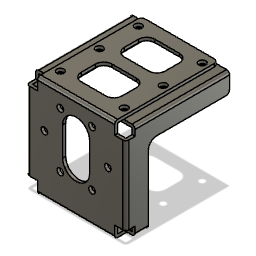
move_base_motor_holder (Autodesk Fusion 360 design; units mm, degrees)
Autodesk Fusion 360 part; units mm, degrees
sketch "スケッチ10" plane through (0, 0, 0) normal (0, 0, 1) x (1, 0, 0)
  line L0 (-18.8, 0) -> (18.8, 0)
  line L1 (18.8, 0) -> (18.8, -4.5)
  line L2 (18.8, -4.5) -> (22.8, -4.5)
  line L3 (22.8, -4.5) -> (22.8, -42.5)
  line L4 (22.8, -42.5) -> (18.8, -42.5)
  line L5 (18.8, -42.5) -> (18.8, -47)
  line L6 (18.8, -47) -> (-18.8, -47)
  line L7 (-18.8, -47) -> (-18.8, -42.5)
  line L8 (-18.8, -42.5) -> (-22.8, -42.5)
  line L9 (-22.8, -42.5) -> (-22.8, -4.5)
  line L10 (-22.8, -4.5) -> (-18.8, -4.5)
  line L11 (-18.8, -4.5) -> (-18.8, 0)
  dimension "d76" = 37.6
  dimension "d77" = 4.5
  dimension "d78" = 38
  dimension "d79" = 4.5
  dimension "d80" = 4
  dimension "d81" = 4
  constraint horizontal L0
  constraint perpendicular L0 L1
  constraint perpendicular L1 L2
  constraint perpendicular L2 L3
  constraint perpendicular L1 L4
  constraint perpendicular L2 L5
  constraint perpendicular L5 L6
  constraint perpendicular L6 L7
  constraint perpendicular L7 L8
  constraint perpendicular L8 L9
  constraint perpendicular L9 L10
  constraint perpendicular L8 L11
  constraint coincident L0.start L11.end
  constraint midpoint origin L0
  constraint collinear L1 L5
  constraint collinear L7 L11
  constraint collinear L2 L10
  constraint collinear L4 L8
  measures "d76" distance of L0.start L0.end
  measures "d77" distance of L0.end L1.end
  measures "d78" distance of L2.end L3.end
  measures "d79" distance of L4.end L5.end
  measures "d80" distance of L1.end L2.end
  measures "d81" distance of L9.end L10.end
extrude "押し出し8" add sketch "スケッチ10" along normal blind 1.5
sketch "スケッチ11" plane through (0, 0, 0) normal (0, 1, 0) x (-1, 0, 0)
  line L0 (-18.8, 0) -> (18.8, 0)
  line L1 (18.8, 0) -> (18.8, 1.5)
  line L2 (18.8, 1.5) -> (-18.8, 1.5)
  line L3 (-18.8, 1.5) -> (-18.8, 0)
  line L4 (18.8, 1.5) -> (-18.8, 1.5)
  line L5 (-18.8, 1.5) -> (-18.8, -49.2)
  line L6 (-18.8, -49.2) -> (18.8, -49.2)
  line L7 (18.8, -49.2) -> (18.8, 1.5)
  line L8 (-10, -7) -> (10, -7)
  line L9 (10, -7) -> (10, -22)
  line L10 (10, -22) -> (-10, -22)
  line L11 (-10, -22) -> (-10, -7)
  line L12 (-10, -28) -> (10, -28)
  line L13 (10, -28) -> (10, -43)
  line L14 (10, -43) -> (-10, -43)
  line L15 (-10, -43) -> (-10, -28)
  point P0 (0, -7)
  dimension "d84" = 50.7
  dimension "d172" = 7
  dimension "d173" = 15
  dimension "d174" = 6
  dimension "d175" = 15
  dimension "d176" = 20
  constraint horizontal L4
  constraint vertical L5
  constraint horizontal L6
  constraint vertical L7
  constraint coincident L1.end L2.start
  constraint coincident L2.end L3.start
  constraint horizontal L8
  constraint vertical L9
  constraint horizontal L10
  constraint vertical L11
  constraint horizontal L12
  constraint vertical L13
  constraint horizontal L14
  constraint vertical L15
  constraint midpoint L8 P0
  constraint collinear L11 L15
  constraint collinear L9 L13
  constraint vertical origin P0
  measures "d84" distance of L2.end L5.end
  measures "d172" distance of origin L8
  measures "d173" distance of L8.end L9.end
  measures "d174" distance of L10 L12
  measures "d175" distance of L12.end L13.end
  measures "d176" distance of L13.end L14.end
extrude "押し出し9" add sketch "スケッチ11" along normal blind 1.5
sketch "スケッチ17" plane through (0, 1.5, 0) normal (0, 1, 0) x (-1, 0, 0)
  line L0 (18.8, -49.2) -> (18.8, 1.5)
  line L1 (18.8, 1.5) -> (-18.8, 1.5)
  line L2 (-18.8, 1.5) -> (-18.8, -49.2)
  line L3 (-18.8, -49.2) -> (18.8, -49.2)
  line L4 (15.6, -6.4) -> (-15.6, -6.4)
  line L5 (-15.6, -6.4) -> (-15.6, -44.5)
  line L6 (-15.6, -44.5) -> (15.6, -44.5)
  line L7 (15.6, -44.5) -> (15.6, -6.4)
  line L8 (15.6, -25.45) -> (-15.6, -25.45)
  line L9 (10, -22) -> (-10, -22)
  line L10 (-10, -22) -> (-10, -7)
  line L11 (-10, -7) -> (10, -7)
  line L12 (10, -7) -> (10, -22)
  line L13 (10, -43) -> (-10, -43)
  line L14 (-10, -43) -> (-10, -28)
  line L15 (-10, -28) -> (10, -28)
  line L16 (10, -28) -> (10, -43)
  point P0 (0, -6.4)
  dimension "d112" = 7.9
  dimension "d113" = 31.2
  dimension "d114" = 19.05
  dimension "d115" = 19.05
  constraint horizontal L4
  constraint vertical L5
  constraint horizontal L6
  constraint vertical L7
  constraint midpoint L4 P0
  constraint vertical origin P0
  constraint coincident L7 L8.start
  constraint coincident L5 L8.end
  constraint perpendicular L5 L8
  measures "d112" distance of L1 L4
  measures "d113" distance of L4.start L4.end
  measures "d114" distance of L4 L8
  measures "d115" distance of L6 L8
hole "穴5" at (-15.6, 1.5, -44.5) at (15.6, 1.5, -44.5) at (15.6, 1.5, -25.45) at (-15.6, 1.5, -25.45) at (-15.6, 1.5, -6.4) at (15.6, 1.5, -6.4) direction (0, -1, 0) diameter 3.5 end through all
sketch "スケッチ12" plane through (0, -47, 0) normal (0, -1, 0) x (1, 0, 0)
  line L0 (-18.8, 0) -> (18.8, 0)
  line L1 (18.8, 0) -> (18.8, 1.5)
  line L2 (18.8, 1.5) -> (-18.8, 1.5)
  line L3 (-18.8, 1.5) -> (-18.8, 0)
  line L4 (18.8, 1.5) -> (-18.8, 1.5)
  line L5 (-18.8, 1.5) -> (-18.8, -9.5)
  line L6 (-18.8, -9.5) -> (18.8, -9.5)
  line L7 (18.8, -9.5) -> (18.8, 1.5)
  dimension "d87" = 11
  constraint horizontal L4
  constraint vertical L5
  constraint horizontal L6
  constraint vertical L7
  constraint coincident L1.end L2.start
  constraint coincident L2.end L3.start
  measures "d87" distance of L4 L6
extrude "押し出し10" add sketch "スケッチ12" along normal blind 1.5
sketch "スケッチ18" plane through (0, -48.5, 0) normal (0, -1, 0) x (1, 0, 0)
  line L0 (18.8, -9.5) -> (18.8, 1.5)
  line L1 (18.8, 1.5) -> (-18.8, 1.5)
  line L2 (-18.8, 1.5) -> (-18.8, -9.5)
  line L3 (-18.8, -9.5) -> (18.8, -9.5)
  line L4 (15.6, -6.4) -> (-15.6, -6.4)
  point P0 (0, -6.4)
  dimension "d119" = 7.9
  dimension "d120" = 31.2
  constraint horizontal L4
  constraint midpoint L4 P0
  constraint vertical origin P0
  measures "d119" distance of L1 L4
  measures "d120" distance of L4.start L4.end
hole "穴6" at (15.6, -48.5, -6.4) at (-15.6, -48.5, -6.4) direction (0, 1, 0) diameter 3.5 depth 1.5 tip angle 118
sketch "スケッチ13" plane through (22.8, 0, 0) normal (1, 0, 0) x (0, 0, -1)
  line L0 (0, -42.5) -> (0, -4.5)
  line L1 (0, -4.5) -> (-1.5, -4.5)
  line L2 (-1.5, -4.5) -> (-1.5, -42.5)
  line L3 (-1.5, -42.5) -> (0, -42.5)
  line L4 (-1.5, -4.5) -> (3, -4.5)
  line L5 (3, -4.5) -> (3, -1.55)
  line L6 (3, -1.55) -> (49.2, -1.55)
  line L7 (9.5, -45.45) -> (3, -45.45)
  line L8 (3, -45.45) -> (3, -42.5)
  line L9 (3, -42.5) -> (-1.5, -42.5)
  line L10 (-1.5, -42.5) -> (-1.5, -4.5)
  line L11 (49.2, -1.55) -> (49.2, -9.5)
  line L12 (49.2, -9.5) -> (9.5, -9.5)
  line L13 (9.5, -9.5) -> (9.5, -45.45)
  dimension "d90" = 4.5
  dimension "d92" = 2.95
  dimension "d93" = 2.95
  dimension "d109" = 46.2
  dimension "d110" = 7.95
  dimension "d111" = 6.5
  constraint coincident L1.end L2.start
  constraint perpendicular L0 L4
  constraint perpendicular L4 L5
  constraint perpendicular L0 L6
  constraint perpendicular L7 L8
  constraint coincident L2.end L3.start
  constraint collinear L5 L8
  constraint perpendicular L6 L11
  constraint perpendicular L11 L12
  constraint perpendicular L12 L13
  constraint coincident L7.start L13.end
  measures "d90" distance of L1.end L4.end
  measures "d92" distance of L4.end L5.end
  measures "d93" distance of L7 L9
  measures "d109" distance of L5.end L6.end
  measures "d110" distance of L6.end L11.end
  measures "d111" distance of L7.start L7.end
extrude "押し出し11" add sketch "スケッチ13" along normal blind 1.5
sketch "スケッチ20" plane through (-22.8, 0, 0) normal (-1, 0, 0) x (0, 0, 1)
  line L0 (0, -4.5) -> (0, -42.5)
  line L1 (0, -42.5) -> (1.5, -42.5)
  line L2 (1.5, -42.5) -> (1.5, -4.5)
  line L3 (1.5, -4.5) -> (0, -4.5)
  line L4 (1.5, -4.5) -> (-3, -4.5)
  line L5 (-3, -4.5) -> (-3, -1.55)
  line L6 (-3, -1.55) -> (-49.2, -1.55)
  line L7 (-49.2, -1.55) -> (-49.2, -9.5)
  line L8 (-49.2, -9.5) -> (-9.5, -9.5)
  line L9 (-9.5, -9.5) -> (-9.5, -45.45)
  line L10 (-9.5, -45.45) -> (-3, -45.45)
  line L11 (-3, -45.45) -> (-3, -42.5)
  line L12 (-3, -42.5) -> (1.5, -42.5)
  line L13 (1.5, -42.5) -> (1.5, -4.5)
  point P0 (-3, -4.5)
  point P1 (-3, -1.55)
  point P2 (-49.2, -1.55)
  point P3 (-49.2, -9.5)
  point P4 (-9.5, -9.5)
  point P5 (-9.5, -45.45)
  point P6 (-3, -42.5)
  constraint coincident L2.end L3.start
  constraint perpendicular L0 L4
  constraint perpendicular L4 L5
  constraint perpendicular L5 L6
  constraint perpendicular L6 L7
  constraint perpendicular L5 L8
  constraint perpendicular L8 L9
  constraint perpendicular L9 L10
  constraint perpendicular L10 L11
  constraint coincident L1.end L2.start
  constraint coincident P0 L4.end
  constraint coincident L6 P1
  constraint coincident P2 L6.end
  constraint coincident P3 L7.end
  constraint coincident L9 P4
  constraint coincident P5 L9.end
  constraint coincident P6 L11.end
extrude "押し出し14" add sketch "スケッチ20" along normal blind 1.5
sketch "スケッチ14" plane through (0, -1.55, 0) normal (0, 1, 0) x (-1, 0, 0)
  line L0 (-22.8, -49.2) -> (-22.8, -3)
  line L1 (-22.8, -3) -> (-24.3, -3)
  line L2 (-24.3, -3) -> (-24.3, -49.2)
  line L3 (-24.3, -3) -> (-11.3, -3)
  line L4 (-11.3, -3) -> (-11.3, -49.2)
  line L5 (-11.3, -49.2) -> (-24.3, -49.2)
  line L6 (-24.3, -49.2) -> (-24.3, -3)
  line L7 (-24.3, -49.2) -> (-22.8, -49.2)
  dimension "d96" = 13
  constraint horizontal L3
  constraint vertical L4
  constraint horizontal L5
  constraint vertical L6
  constraint coincident L1.end L2.start
  constraint coincident L2.end L5.end
  measures "d96" distance of L4.end L2.end
extrude "押し出し12" add sketch "スケッチ14" along normal blind 1.5
sketch "スケッチ19" plane through (0, -0.05, 0) normal (0, 1, 0) x (-1, 0, 0)
  line L0 (-11.3, -49.2) -> (-11.3, -3)
  line L1 (-11.3, -3) -> (-24.3, -3)
  line L2 (-24.3, -3) -> (-24.3, -49.2)
  line L3 (-24.3, -49.2) -> (-11.3, -49.2)
  line L4 (-15.6, -6.4) -> (-15.6, -44.5)
  line L5 (18.8, 1.5) -> (-18.8, 1.5)
  point P0 (-15.6, -25.45)
  dimension "d124" = 15.6
  dimension "d125" = 7.9
  dimension "d126" = 38.1
  constraint parallel L0 L4
  constraint midpoint L4 P0
  measures "d124" distance of origin L4
  measures "d125" distance of L4.start L5
  measures "d126" distance of L4.start L4.end
hole "穴7" at (15.6, -0.05, -44.5) at (15.6, -0.05, -25.45) at (15.6, -0.05, -6.4) direction (0, -1, 0) diameter 3 depth 1.5 tip angle 118
sketch "スケッチ15" plane through (0, -45.45, 0) normal (0, -1, 0) x (1, 0, 0)
  line L0 (22.8, -3) -> (22.8, -9.5)
  line L1 (24.3, -9.5) -> (24.3, -3)
  line L2 (24.3, -3) -> (22.8, -3)
  line L3 (24.3, -3) -> (11.3, -3)
  line L4 (11.3, -3) -> (11.3, -9.5)
  line L5 (11.3, -9.5) -> (24.3, -9.5)
  line L6 (24.3, -9.5) -> (24.3, -3)
  line L7 (22.8, -9.5) -> (24.3, -9.5)
  line L8 (18.8, 1.5) -> (-18.8, 1.5)
  point P0 (15.6, -6.4)
  dimension "d99" = 13
  dimension "d134" = 7.9
  dimension "d135" = 15.6
  constraint horizontal L3
  constraint vertical L4
  constraint horizontal L5
  constraint vertical L6
  constraint coincident L1.end L2.start
  constraint coincident L1.start L5.end
  measures "d99" distance of L4 L6
  measures "d134" distance of P0 L8
  measures "d135" horizontal distance of origin P0
extrude "押し出し13" add sketch "スケッチ15" along normal blind 1.5
hole "穴8" at (15.6, -45.45, -6.4) direction (0, -1, 0) diameter 3 end through all
sketch "スケッチ21" plane through (0, -1.55, 0) normal (0, 1, 0) x (-1, 0, 0)
  line L0 (22.8, -3) -> (22.8, -49.2)
  line L1 (22.8, -49.2) -> (24.3, -49.2)
  line L2 (24.3, -49.2) -> (24.3, -3)
  line L3 (24.3, -3) -> (22.8, -3)
  line L4 (24.3, -3) -> (11.3, -3)
  line L5 (11.3, -3) -> (11.3, -49.2)
  line L6 (11.3, -49.2) -> (24.3, -49.2)
  line L7 (24.3, -49.2) -> (24.3, -3)
  line L8 (15.6, -6.4) -> (15.6, -44.5)
  line L9 (18.8, 1.5) -> (-18.8, 1.5)
  point P0 (15.6, -25.45)
  dimension "d139" = 13
  dimension "d140" = 7.9
  dimension "d141" = 15.6
  dimension "d142" = 38.1
  constraint horizontal L4
  constraint vertical L5
  constraint horizontal L6
  constraint vertical L7
  constraint coincident L2.end L3.start
  constraint coincident L1.end L2.start
  constraint vertical L8
  constraint midpoint L8 P0
  measures "d139" distance of L5 L7
  measures "d140" distance of L8.start L9
  measures "d141" horizontal distance of origin L8.start
  measures "d142" distance of L8.start L8.end
extrude "押し出し15" add sketch "スケッチ21" along normal blind 1.5
hole "穴9" at (-15.6, -1.55, -44.5) at (-15.6, -1.55, -25.45) at (-15.6, -1.55, -6.4) direction (0, 1, 0) diameter 3 end through all
sketch "スケッチ22" plane through (0, -45.45, 0) normal (0, -1, 0) x (1, 0, 0)
  line L0 (-22.8, -9.5) -> (-22.8, -3)
  line L1 (-22.8, -3) -> (-24.3, -3)
  line L2 (-24.3, -3) -> (-24.3, -9.5)
  line L3 (-24.3, -9.5) -> (-22.8, -9.5)
  line L4 (-24.3, -3) -> (-11.3, -3)
  line L5 (-11.3, -3) -> (-11.3, -9.5)
  line L6 (-11.3, -9.5) -> (-24.3, -9.5)
  line L7 (-24.3, -9.5) -> (-24.3, -3)
  line L8 (18.8, 1.5) -> (-18.8, 1.5)
  point P0 (-15.6, -6.4)
  dimension "d148" = 13
  dimension "d149" = 7.9
  dimension "d150" = 15.6
  constraint horizontal L4
  constraint vertical L5
  constraint horizontal L6
  constraint vertical L7
  constraint coincident L1.end L2.start
  constraint coincident L2.end L3.start
  measures "d148" distance of L5 L7
  measures "d149" distance of P0 L8
  measures "d150" horizontal distance of origin P0
extrude "押し出し16" add sketch "スケッチ22" along normal blind 1.5
hole "穴10" at (-15.6, -45.45, -6.4) direction (0, -1, 0) diameter 3 end through all
thread "ねじ1" "ISO Metric profile 3.0 M3x0.5 6H" major diameter 3.086 minor diameter 2.529 pitch 0.5 angle 60 resizes the face on face at (15.7494, -1.05, -4.9075) on face at (16.9348, -1.05, -45.1843) on face at (-14.2327, -1.05, -43.8831) on face at (15.7494, -1.05, -23.9575) on face at (-15.4506, -0.55, -7.8925) on face at (-15.5252, -1.05, -26.9481) on face at (15.7494, -46.45, -4.9075) on face at (-15.4506, -46.45, -4.9075)
fillet "フィレット3" radius 1.5 8 edges at (0, 1.5, 1.5) (-24.3, -0.05, -26.1) (24.3, -0.05, -26.1) (24.3, -23.5, 1.5) (-24.3, -23.5, 1.5) (0, -48.5, 1.5) (-24.3, -46.95, -6.25) (24.3, -46.95, -6.25)
sketch "スケッチ23" plane through (0, 0, 1.5) normal (0, 0, 1) x (1, 0, 0)
  line L0 (-18.8, -47) -> (18.8, -47)
  line L1 (18.8, -47) -> (18.8, -42.5)
  line L2 (18.8, -42.5) -> (22.8, -42.5)
  line L3 (22.8, -42.5) -> (22.8, -4.5)
  line L4 (22.8, -4.5) -> (18.8, -4.5)
  line L5 (18.8, -4.5) -> (18.8, 0)
  line L6 (18.8, 0) -> (-18.8, 0)
  line L7 (-18.8, 0) -> (-18.8, -4.5)
  line L8 (-18.8, -4.5) -> (-22.8, -4.5)
  line L9 (-22.8, -4.5) -> (-22.8, -42.5)
  line L10 (-22.8, -42.5) -> (-18.8, -42.5)
  line L11 (-18.8, -42.5) -> (-18.8, -47)
  circle A0 centre (0, -19.8) radius 15.5
  line L12 (-15.5, -19.8) -> (15.5, -19.8)
  line L13 (-7.75, -6.3766) -> (7.75, -33.2234)
  line L14 (7.75, -6.3766) -> (-7.75, -33.2234)
  line L15 (-6.6, -12.8) -> (6.6, -12.8)
  line L16 (6.6, -12.8) -> (6.6, -26.8)
  line L17 (6.6, -26.8) -> (-6.6, -26.8)
  line L18 (-6.6, -26.8) -> (-6.6, -12.8)
  line L19 (-6.6, -12.8) -> (6.6, -26.8) construction
  line L20 (6.6, -12.8) -> (-6.6, -26.8) construction
  circle A1 centre (0, -12.8) radius 6.6
  circle A2 centre (0, -26.8) radius 6.6
  point P0 (0, -19.8)
  dimension "d158" = 19.8
  dimension "d159" = 31
  dimension "d160" = 60
  dimension "d161" = 60
  dimension "d162" = 14
  dimension "d163" = 13.2
  constraint vertical origin A0.centre
  constraint coincident A0 L12.start
  constraint coincident A0 L12.end
  constraint horizontal L12
  constraint coincident A0 L13.start
  constraint coincident A0 L13.end
  constraint coincident A0 L14.start
  constraint coincident A0 L14.end
  constraint midpoint P0 L12
  constraint midpoint P0 L13
  constraint midpoint P0 L14
  constraint horizontal L15
  constraint perpendicular L15 L16
  constraint parallel L15 L17
  constraint parallel L16 L18
  constraint coincident L19 P0
  constraint coincident L20 P0
  constraint coincident P0 A0.centre
  constraint midpoint L15 A1.centre
  constraint midpoint L17 A2.centre
  constraint tangent L16 A1
  constraint tangent L16 A2
  measures "d158" distance of origin A0.centre
  measures "d159" diameter of A0
  measures "d160" angle of L12 L14
  measures "d161" angle of L12 L13
  measures "d162" distance of L15.start L17.end
  measures "d163" diameter of A1
extrude "押し出し17" cut sketch "スケッチ23" against normal through all contours L12 L13 L16 A2 | L12 L14 L16 A1 | L14 L15 A1 | L13 L14 L15 A1 | L13 L14 L17 A2 | L13 L17 A2 | L12 L14 L18 A2 | L12 L13 L18 A1 | L13 L14 A1 | L13 L14 A2 | L14 L15 A1 | L13 L17 A2 | L13 L15 A1 | L13 L14 L15 A1 | L14 L17 A2 | L13 L14 L17 A2 | L13 L15 A1 | L14 L17 A2
hole "穴11" at (7.75, -6.3766, 1.5) at (-7.75, -6.3766, 1.5) at (-15.5, -19.8, 1.5) at (-7.75, -33.2234, 1.5) at (7.75, -33.2234, 1.5) at (15.5, -19.8, 1.5) direction (0, 0, -1) diameter 3.2 end through all
fillet "フィレット4" radius 2 14 edges at (18.8, 0.75, -49.2) (-18.8, 0.75, -49.2) (-11.3, -0.8, -49.2) (11.3, -0.8, -49.2) (23.55, -9.5, -49.2) (-23.55, -9.5, -49.2) (18.8, -47.75, -9.5) (11.3, -46.2, -9.5) (-11.3, -46.2, -9.5) (-18.8, -47.75, -9.5) (11.3, -0.8, -3) (-11.3, -0.8, -3) (-11.3, -46.2, -3) (11.3, -46.2, -3)
fillet "フィレット5" radius 4 2 edges at (23.55, -9.5, -9.5) (-23.55, -9.5, -9.5)
fillet "フィレット6" radius 4 8 edges at (10, 0.75, -7) (-10, 0.75, -7) (-10, 0.75, -22) (10, 0.75, -22) (10, 0.75, -28) (-10, 0.75, -28) (10, 0.75, -43) (-10, 0.75, -43)
